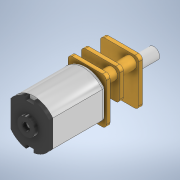
# Autodesk Inventor part: GA12-N20微型减速直流电机3V_15RPM
Saved by Autodesk Inventor 2022 (Build 260153000, 153)
## iProperties
Created: 2022-05-21
Part Number: GA12-N20微型减速直流电机3V_15RPM
Material: 常规
Document SubType Name: Modeling
Designer: zhcne
Density: 1 g/cm^3
Appearance: 默认
Author: zhcne
Autodesk Inventor part; units mm, degrees
ref_plane "YZ Plane" through (0, 0, 0) normal (1, 0, 0) x (0, 1, 0)
ref_plane "XZ Plane" through (0, 0, 0) normal (0, 1, 0) x (-1, 0, 0)
ref_plane "XY Plane" through (0, 0, 0) normal (0, 0, 1) x (1, 0, 0)
sketch "草图1" plane through (0, 0, 0) normal (0, 0, 1) x (1, 0, 0)
  circle A0 centre (0, 0) radius 2.25
  circle A1 centre (0, 0) radius 1
  dimension "d0" = 4.5
  dimension "d1" = 2
  constraints: 2 centre point, 2 coincident
  measures "d0" diameter of A0
  measures "d1" diameter of A1
extrude "拉伸1" add sketch "草图1" against normal blind 1
sketch "草图2" plane through (0, 0, -1) normal (0, 0, -1) x (-1, 0, 0)
  line L0 (5, 3.5) -> (5, -3.5)
  line L1 (-5, 3.5) -> (-5, -3.5)
  line L2 (5, -3.5) -> (-5, -3.5) construction
  line L3 (5, 3.5) -> (-5, 3.5) construction
  line L4 (0, 0) -> (0, 19.9498)
  line L5 (0, 0) -> (7.1401, 0)
  line L6 (1, 5.9195) -> (1, 5)
  line L7 (1, 5) -> (-1, 5)
  line L8 (-1, 5) -> (-1, 5.9195)
  arc A0 (5, 3.5) -> (1, 5.9195) centre (0, -0.25) ccw
  arc A1 (-1, 5.9195) -> (-5, 3.5) centre (0, -0.25) ccw
  line L9 (1, -5.9195) -> (1, -5)
  line L10 (1, -5) -> (-1, -5)
  line L11 (-1, -5) -> (-1, -5.9195)
  arc A2 (-5, -3.5) -> (-1, -5.9195) centre (0, 0.25) ccw
  arc A3 (1, -5.9195) -> (5, -3.5) centre (0, 0.25) ccw
  point P0 (0, 6)
  point P1 (0, 6)
  dimension "d4" = 10
  dimension "d7" = 7
  dimension "d8" = 6
  dimension "d9" = 1
  dimension "d10" = 2
  constraints: 24 end point, 9 point on circle, 5 symmetric about line, 4 centre point, 4 vertical, 3 horizontal, 2 perpendicular, 1 coincident, 1 point on line, 3 other
  measures "d4" distance between parallel lines of L1 L0
  measures "d7" distance of L0.start L0.end
  measures "d8" distance of L4.start point (0, 6)
  measures "d9" distance from line of L7 point (0, 6)
  measures "d10" distance between parallel lines of L8 L6
extrude "拉伸2" add sketch "草图2" along normal blind 1
sketch "草图3" plane through (0, 0, -2) normal (0, 0, -1) x (-1, 0, 0)
  line L0 (1, 5) -> (-1, 5) construction
  line L1 (-1, 5) -> (-1, 5.9195) construction
  arc A0 (-1, 5.9195) -> (-5, 3.5) centre (0, -0.25) ccw construction
  line L2 (-5, 3.5) -> (-5, -3.5) projected
  arc A1 (-5, -3.5) -> (-1, -5.9195) centre (0, 0.25) ccw construction
  line L3 (-1, -5.9195) -> (-1, -5) construction
  line L4 (-1, -5) -> (1, -5) construction
  line L5 (1, -5) -> (1, -5.9195) construction
  arc A2 (1, -5.9195) -> (5, -3.5) centre (0, 0.25) ccw construction
  line L6 (5, -3.5) -> (5, 3.5) projected
  arc A3 (5, 3.5) -> (1, 5.9195) centre (0, -0.25) ccw construction
  line L7 (1, 5.9195) -> (1, 5) construction
  arc A4 (5, 3.5) -> (-5, 3.5) centre (0, -0.25) ccw
  line L8 (0, 0) -> (3.3982, 0)
  arc A5 (-5, -3.5) -> (5, -3.5) centre (0, 0.25) ccw
  constraints: 4 end point, 4 point on circle, 2 centre point, 1 coincident, 1 horizontal, 1 symmetric about line, 1 other
extrude "拉伸3" add sketch "草图3" along normal blind 14 separate body
fillet "圆角1" radius 1 4 edges at (0, 6, -16) (-5, 0, -16) (0, -6, -16) (5, 0, -16)
sketch "草图4" plane through (0, 0, -16) normal (0, 0, -1) x (-1, 0, 0)
  line L0 (-5, 5) -> (-5, -5)
  line L1 (-4, -6) -> (4, -6)
  line L2 (5, -5) -> (5, 5)
  line L3 (4, 6) -> (-4, 6)
  line L4 (0, 0) -> (0, 19.5528)
  line L5 (0, 0) -> (-9.7016, 0)
  arc A0 (-5, -5) -> (-4, -6) centre (-4, -5) ccw
  arc A1 (-4, 6) -> (-5, 5) centre (-4, 5) ccw
  arc A2 (5, 5) -> (4, 6) centre (4, 5) ccw
  arc A3 (4, -6) -> (5, -5) centre (4, -5) ccw
  dimension "d16" = 1
  dimension "d17" = 10
  dimension "d18" = 12
  constraints: 12 end point, 8 point on circle, 8 tangent, 4 centre point, 3 equal radius, 3 perpendicular, 2 vertical, 1 horizontal, 2 other
  measures "d16" radius of A0
  measures "d17" distance between parallel lines of L2 L0
  measures "d18" distance between parallel lines of L1 L3
extrude "拉伸4" add sketch "草图4" along normal blind 1 separate body
sketch "草图5" plane through (0, 0, -17) normal (0, 0, -1) x (-1, 0, 0)
  circle A0 centre (3, -4) radius 1.5
  circle A1 centre (-3, 4) radius 1.5
  line L0 (5, -5) -> (5, 5) projected
  line L1 (-4, -6) -> (4, -6) projected
  line L2 (4, 6) -> (-4, 6) projected
  line L3 (-5, 5) -> (-5, -5) projected
  point P0 (0, 0)
  dimension "d21" = 3
  dimension "d22" = 2
  dimension "d23" = 2
  dimension "d24" = 2
  dimension "d25" = 2
  constraints: 2 centre point, 1 equal radius
  measures "d21" diameter of A1
  measures "d22" distance from line of L0 A0.centre
  measures "d23" distance from line of L1 A0.centre
  measures "d24" distance from line of L2 A1.centre
  measures "d25" distance from line of L3 A1.centre
extrude "拉伸5" add sketch "草图5" along normal blind 2.5 bodies 3
sketch "草图6" plane through (-3, -4, -19.5) normal (0, 0, -1) x (-1, 0, 0)
  circle A0 centre (-6, 8) radius 1.5 construction
  circle A1 centre (0, 0) radius 1.5 construction
  line L0 (-8, 9) -> (-8, -1) projected
  arc A2 (-8, -1) -> (-7, -2) centre (-7, -1) ccw projected
  line L1 (-7, -2) -> (1, -2) projected
  arc A3 (1, -2) -> (2, -1) centre (1, -1) ccw projected
  line L2 (2, -1) -> (2, 9) projected
  arc A4 (2, 9) -> (1, 10) centre (1, 9) ccw projected
  line L3 (1, 10) -> (-7, 10) projected
  arc A5 (-7, 10) -> (-8, 9) centre (-7, 9) ccw projected
  point P0 (-3, 4)
extrude "拉伸6" add sketch "草图6" along normal blind 1 bodies 3
sketch "草图7" plane through (-3, -4, -20.5) normal (0, 0, -1) x (-1, 0, 0)
  circle A0 centre (0, 0) radius 1.5 projected
  circle A1 centre (-6, 8) radius 1.5 projected
  point P0 (-3, 4)
extrude "拉伸7" add sketch "草图7" along normal blind 4 bodies 3
sketch "草图8" plane through (-3, -4, -24.5) normal (0, 0, -1) x (-1, 0, 0)
  circle A0 centre (-6, 8) radius 1.5 construction
  circle A1 centre (0, 0) radius 1.5 construction
  arc A2 (-8, -1) -> (-7, -2) centre (-7, -1) ccw projected
  line L0 (-7, -2) -> (1, -2) projected
  arc A3 (1, -2) -> (2, -1) centre (1, -1) ccw projected
  line L1 (2, -1) -> (2, 9) projected
  arc A4 (2, 9) -> (1, 10) centre (1, 9) ccw projected
  line L2 (1, 10) -> (-7, 10) projected
  arc A5 (-7, 10) -> (-8, 9) centre (-7, 9) ccw projected
  line L3 (-8, 9) -> (-8, -1) projected
  point P0 (-3, 4)
extrude "拉伸8" add sketch "草图8" along normal blind 1 bodies 3
sketch "草图9" plane through (-3, -4, -25.5) normal (0, 0, -1) x (-1, 0, 0)
  circle A0 centre (-3, 4) radius 1 projected
  circle A1 centre (-3, 4) radius 2
  circle A2 centre (-3, 4) radius 1.5
  dimension "d34" = 4
  dimension "d35" = 3
  constraints: 2 centre point, 2 coincident
  measures "d34" diameter of A1
  measures "d35" diameter of A2
extrude "拉伸9" add sketch "草图9" along normal blind 0.5 contours A1 bodies 3
sketch "草图10" plane through (0, 0, -25.5) normal (0, 0, -1) x (-1, 0, 0)
  circle A0 centre (0, 0) radius 1.5
  circle A1 centre (0, 0) radius 1.5 projected
  line L0 (1.2689, -0.8) -> (-1.2689, -0.8)
  point P0 (1.2689, -0.8)
  dimension "d38" = 2.3
  dimension "d39" = 3
  constraints: 2 end point, 2 point on circle, 1 centre point, 1 coincident, 1 horizontal
  measures "d39" diameter of A0
sketch "草图11" plane through (-3, -4, -20.5) normal (0, 0, -1) x (-1, 0, 0)
  line L0 (-7, 2) -> (-4, 2)
  line L1 (-4, 2) -> (-4, -1)
  line L2 (-7, -2) -> (1, -2) construction
  line L3 (-7, -2) -> (1, -2) projected
  arc A0 (-4, -1) -> (-3, -2) centre (-3, -1) ccw
  arc A1 (-8, 3) -> (-7, 2) centre (-7, 3) ccw
  arc A2 (-8, -1) -> (-7, -2) centre (-7, -1) ccw projected
  line L4 (-3, -2) -> (-7, -2)
  arc A3 (-8, 0.5) -> (2, 0.5) centre (-3, 4.25) ccw construction
  line L5 (-8, 9) -> (-8, -1) construction
  line L6 (-8, 3) -> (-8, -1)
  point P0 (-3, 4)
  point P1 (-8, 2)
  point P2 (-4, -2)
  dimension "d45" = 4
  dimension "d46" = 1
  dimension "d47" = 1
  constraints: 8 end point, 5 tangent, 4 point on circle, 3 point on line, 2 centre point, 2 horizontal, 1 perpendicular, 1 vertical
  measures "d45" distance between parallel lines of L2 L0
  measures "d46" radius of A0
  measures "d47" radius of A1
extrude "拉伸12" cut sketch "草图11" against normal blind 1.5 bodies 3
extrude "拉伸10" add sketch "草图10" along normal blind 0.6 bodies 3
extrude "拉伸13" add sketch "草图10" along normal blind 8 contours A0 L0 picked at (0.3589, -0.0009) bodies 3
